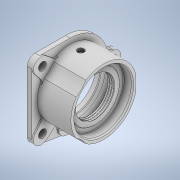
# Autodesk Inventor part: 72. Крышка подшипника
Saved by Autodesk Inventor 2021 (Build 250183000, 183)
## iProperties
Created: 2021-03-26
Part Number: 72. Крышка подшипника
Material: Типовые
Document SubType Name: Modeling
Designer: Данил
Density: 1 g/cm^3
Appearance: По умолчанию
Author: Данил
Autodesk Inventor part; units mm, degrees
ref_plane "XY Plane" through (0, 0, 0) normal (0, 0, 1) x (1, 0, 0)
sketch "Эскиз1" plane through (0, 0, 0) normal (0, 0, 1) x (1, 0, 0)
  line L0 (-25, 0) -> (25, 0)
  line L1 (25, -43) -> (25, -39.1547)
  line L2 (23, -38) -> (13.8, -38)
  line L3 (25, -43) -> (-15.3397, -43)
  line L4 (23, -38) -> (25, -39.1547)
  line L5 (13, -37.2) -> (13, -31.5)
  line L6 (13, -31.5) -> (14, -31.5)
  line L7 (14, -31.5) -> (14, -25.5)
  line L8 (14, -25.5) -> (5, -25.5)
  arc A0 (13, -37.2) -> (13.8, -38) centre (13.8, -37.2) ccw
  line L9 (5, -25.5) -> (5, -35)
  line L10 (2, -38) -> (-11, -38)
  arc A1 (2, -38) -> (5, -35) centre (2, -35) ccw
  line L11 (-14, -35) -> (-20, -35)
  line L12 (-20.5, -35.5) -> (-20.5, -39.5)
  line L13 (-21, -40) -> (-23, -40)
  arc A2 (-21, -40) -> (-20.5, -39.5) centre (-21, -39.5) ccw
  arc A3 (-20, -35) -> (-20.5, -35.5) centre (-20, -35.5) ccw
  line L14 (-23, -40) -> (-23, -43)
  line L15 (-23.5, -43.5) -> (-25, -43.5)
  arc A4 (-23.5, -43.5) -> (-23, -43) centre (-23.5, -43) ccw
  arc A5 (-14, -35) -> (-11, -38) centre (-11, -35) ccw
  point P0 (0, 0)
  point P1 (0, 0)
  point P2 (25, -38)
  dimension "d0" = 50
  dimension "d1" = 86
  dimension "d2" = 2
  dimension "d3" = 30
  dimension "d4" = 76
  dimension "d5" = 0.8
  dimension "d6" = 11
  dimension "d7" = 1
  dimension "d8" = 63
  dimension "d9" = 51
  dimension "d10" = 30
  dimension "d11" = 3
  dimension "d12" = 76
  dimension "d16" = 4.5
  dimension "d17" = 0.5
  dimension "d18" = 0.5
  dimension "d19" = 80
  dimension "d20" = 87
  dimension "d21" = 2
  dimension "d22" = 70
  dimension "d23" = 3
  dimension "d24" = 11
  constraints: 32 end point, 12 point on circle, 10 tangent, 6 centre point, 6 perpendicular, 5 vertical, 4 horizontal, 3 vertical alignment, 2 point on line, 1 coincident, 1 equal radius, 1 midpoint
  measures "d0" distance of L0.start L0.end
  measures "d1" diameter of L3 L0
  measures "d2" distance of L2.start point (25, -38)
  measures "d3" angle of L2 L4
  measures "d4" diameter of L2 L0
  measures "d5" radius of A0
  measures "d6" distance from line of L0.end L7
  measures "d7" distance between parallel lines of L7 L5
  measures "d8" diameter of L6 L0
  measures "d9" diameter of L8 L0
  measures "d10" distance from line of L0.start L9
  measures "d11" radius of A1
  measures "d12" diameter of L10 L0
  measures "d16" distance from line of L0.start L12
  measures "d17" radius of A2
  measures "d18" radius of A4
  measures "d19" diameter of L13 L0
  measures "d20" diameter of L15 L0
  measures "d21" distance from line of L0.start L14
  measures "d22" diameter of L11 L0
  measures "d23" radius of A5
  measures "d24" horizontal distance of L0.start L11.start
ref_plane "РабПлоскость1" through (-25, 0, 0) normal (1, 0, 0) x (0, 1, 0)
sketch "Эскиз2" plane through (-25, 0, 0) normal (1, 0, 0) x (0, 1, 0)
  circle A0 centre (0, 0) radius 54 construction
  arc A1 (16.522, -47.1914) -> (9.9132, -55.3148) centre (19.8264, -56.6296) ccw
  arc A2 (-9.9132, -55.3148) -> (9.9132, -55.3148) centre (0, -54) ccw
  arc A3 (-9.9132, -55.3148) -> (-16.522, -47.1914) centre (-19.8264, -56.6296) ccw
  circle A4 centre (0, -54) radius 5.25
  line L0 (50, 0) -> (50, 40)
  arc A5 (50, 40) -> (40, 50) centre (40, 40) ccw
  line L1 (40, 50) -> (-40, 50)
  line L2 (0, 0) -> (40, 40) construction
  line L3 (0, 0) -> (0, 54) construction
  circle A6 centre (38.1838, 38.1838) radius 5.25
  arc A7 (16.522, -47.1914) -> (50, 0) centre (0, 0) ccw
  arc A8 (-40, 50) -> (-49.8662, 41.6305) centre (-40, 40) ccw
  line L4 (0, 0) -> (-40, 40) construction
  circle A9 centre (-38.1838, 38.1838) radius 5.25
  line L5 (-49.8662, 41.6305) -> (-55.4149, 8.0564)
  arc A10 (-55.4149, 8.0564) -> (-54.7664, 2.1552) centre (-44.5621, 6.2628) ccw
  line L6 (-54.7664, 2.1552) -> (-46.3832, -18.6708)
  line L7 (0, 0) -> (-54, 0) construction
  line L8 (0, 0) -> (-44.5621, 6.2628) construction
  arc A11 (-46.3832, -18.6708) -> (-16.522, -47.1914) centre (0, 0) ccw
  circle A12 centre (0, 0) radius 45 construction
  dimension "d44" = 90
  dimension "d28" = 108
  dimension "d29" = 10
  dimension "d30" = 10.5
  dimension "d32" = 10
  dimension "d33" = 45
  dimension "d34" = 10.5
  dimension "d35" = 50
  dimension "d37" = 45
  dimension "d38" = 10.5
  dimension "d39" = 11
  dimension "d40" = 10
  dimension "d41" = 8
  dimension "d43" = 50
  constraints: 21 point on circle, 18 end point, 12 centre point, 12 tangent, 4 coincident, 2 equal radius, 2 point on line, 2 vertical alignment, 1 horizontal, 1 perpendicular, 1 vertical, 3 other
  measures "d28" diameter of A0
  measures "d29" radius of A2
  measures "d30" diameter of A4
  measures "d32" radius of A5
  measures "d33" angle of L3 L2
  measures "d34" diameter of A6
  measures "d35" radius of A7
  measures "d37" angle of L4 L3
  measures "d38" diameter of A9
  measures "d39" radius of A10
  measures "d40" radius of A8
  measures "d41" angle of L8 L7
  measures "d43" radius of A11
extrude "Выдавливание1" add sketch "Эскиз2" along normal blind 6
sketch "Эскиз3" plane through (-19, 0, 0) normal (1, 0, 0) x (0, 0, -1)
  arc A0 (55.3148, -9.9132) -> (55.3148, 9.9132) centre (54, 0) ccw projected
  arc A1 (55.3148, -9.9132) -> (47.1914, -16.522) centre (56.6296, -19.8264) ccw projected
  circle A2 centre (0, 0) radius 43
  line L0 (55.3148, 9.9132) -> (41.3595, 11.7641)
  line L1 (55.3148, -9.9132) -> (41.3595, -11.7641)
  arc A3 (-50, -40) -> (-41.6305, -49.8662) centre (-40, -40) ccw projected
  arc A4 (-47.8134, -33.759) -> (-33.759, -47.8134) centre (-40, -40) ccw
  line L2 (-33.759, -47.8134) -> (-20.9272, -37.564)
  line L3 (-47.8134, -33.759) -> (-37.564, -20.9272)
  line L4 (-37.564, -20.9272) -> (-20.9272, -37.564) construction
  line L5 (0, 0) -> (0, -43) construction
  line L6 (0, 0) -> (-29.2456, -29.2456) construction
  arc A5 (-40, 50) -> (-50, 40) centre (-40, 40) ccw projected
  arc A6 (-33.759, 47.8134) -> (-47.8134, 33.759) centre (-40, 40) ccw
  line L7 (-33.759, 47.8134) -> (-20.9272, 37.564)
  line L8 (-47.8134, 33.759) -> (-37.564, 20.9272)
  line L9 (-37.564, 20.9272) -> (-20.9272, 37.564) construction
  line L10 (0, 0) -> (-29.2456, 29.2456) construction
  circle A7 centre (-38.1838, 38.1838) radius 5.25 projected
  circle A8 centre (54, 0) radius 5.25 projected
  circle A9 centre (-38.1838, -38.1838) radius 5.25 projected
  arc A10 (-8.0564, -55.4149) -> (-2.1552, -54.7664) centre (-6.2628, -44.5621) ccw projected
  arc A11 (-17.2628, -44.5621) -> (4.4747, -42.1733) centre (-6.2628, -44.5621) ccw
  line L11 (-17.2628, -44.5621) -> (-17.2628, -39.3827)
  point P0 (-41.6305, -49.8662)
  point P1 (-5.0612, -55.4962)
  point P2 (-8.0564, -55.4149)
  point P3 (-2.1552, -54.7664)
  point P4 (4.5877, -42.7546)
  dimension "d47" = 86
  dimension "d48" = 45
  dimension "d49" = 23.528
  dimension "d50" = 90
  dimension "d51" = 23.528
  constraints: 24 end point, 8 point on circle, 7 tangent, 4 coincident, 3 centre point, 2 concentric, 2 midpoint, 2 vertical, 10 other
  measures "d48" angle of L5 L6
  measures "d49" distance of L3.end L2.end
  measures "d50" angle of L6 L10
  measures "d51" distance of L8.end L7.end
extrude "Выдавливание2" add sketch "Эскиз3" along normal blind 2 contours L1 A2 L0 A0 | A11 A10 L11 A2 | A2 L8 A6 A5 L7 | L2 A4 A3 L3 A2
sketch "Эскиз4" plane through (0, 0, 0) normal (0, 0, 1) x (1, 0, 0)
  line L0 (-25, 0) -> (25, 0)
  line L1 (25, -43) -> (-23, -43)
  line L2 (25, -43) -> (25, -39.1547)
  line L3 (25, -39.1547) -> (23, -38)
  line L4 (23, -38) -> (13.8, -38)
  line L5 (13, -37.2) -> (13, -32.3)
  line L6 (13.8, -31.5) -> (14, -31.5)
  line L7 (14, -31.5) -> (14, -25.5)
  line L8 (14, -25.5) -> (5, -25.5)
  arc A0 (13, -37.2) -> (13.8, -38) centre (13.8, -37.2) ccw
  arc A1 (13.8, -31.5) -> (13, -32.3) centre (13.8, -32.3) ccw
  line L9 (5, -25.5) -> (5, -35)
  line L10 (2, -38) -> (-11, -38)
  line L11 (-14, -35) -> (-14, -35)
  arc A2 (2, -38) -> (5, -35) centre (2, -35) ccw
  arc A3 (-13.9047, -35.75) -> (-11, -38) centre (-11, -35) ccw
  line L12 (-14.873, -35) -> (-20.5, -35)
  arc A4 (-13.9047, -35.75) -> (-14.873, -35) centre (-14.873, -36) ccw
  line L13 (-20.5, -35) -> (-20.5, -39.5)
  line L14 (-21, -40) -> (-23, -40)
  arc A5 (-21, -40) -> (-20.5, -39.5) centre (-21, -39.5) ccw
  line L15 (-23, -40) -> (-23, -43)
  line L16 (-23.5, -43.5) -> (-25, -43.5)
  arc A6 (-23.5, -43.5) -> (-23, -43) centre (-23.5, -43) ccw
  point P0 (0, 0)
  point P1 (0, 0)
  dimension "d54" = 50
  dimension "d55" = 86
  dimension "d56" = 30
  dimension "d57" = 2
  dimension "d58" = 76
  dimension "d59" = 51
  dimension "d60" = 1
  dimension "d61" = 11
  dimension "d62" = 0.8
  dimension "d63" = 63
  dimension "d64" = 30
  dimension "d65" = 3
  dimension "d66" = 76
  dimension "d67" = 11
  dimension "d68" = 70
  dimension "d69" = 1
  dimension "d70" = 4.5
  dimension "d71" = 0.5
  dimension "d72" = 80
  dimension "d73" = 87
  dimension "d74" = 0.5
  dimension "d75" = 2
  constraints: 34 end point, 15 point on circle, 14 tangent, 7 centre point, 6 perpendicular, 5 horizontal, 5 vertical, 2 coincident, 2 equal radius, 2 vertical alignment, 1 midpoint, 1 point on line
  measures "d54" distance of L0.start L0.end
  measures "d55" diameter of L1.start L0
  measures "d56" angle of L4 L3
  measures "d57" horizontal distance of L3.end L2.end
  measures "d58" diameter of L4 L0
  measures "d59" diameter of L8 L0
  measures "d60" distance between parallel lines of L7 L5
  measures "d61" distance from line of L0.end L7
  measures "d62" radius of A0
  measures "d63" diameter of L6 L0
  measures "d64" horizontal distance of L0.start L8.end
  measures "d65" radius of A2
  measures "d66" diameter of L10 L0
  measures "d67" distance from line of L0.start L11
  measures "d68" diameter of L12 L0
  measures "d69" radius of A4
  measures "d70" distance from line of L0.start L13
  measures "d71" radius of A5
  measures "d72" diameter of L14.end L0
  measures "d73" diameter of L16.end L0
  measures "d74" radius of A6
  measures "d75" distance from line of L16.end L15
revolve "Вращение1" add sketch "Эскиз4" angle 360 about axis through (-25, 0, 0) along (1, 0, 0)
sketch "Эскиз5" plane through (0, 0, 0) normal (0, 0, 1) x (1, 0, 0)
  line L0 (-23.5, -43.5) -> (-25, -43.5) projected
  arc A0 (-23.5, -43.5) -> (-23, -43) centre (-23.5, -43) ccw projected
  line L1 (-23, -40) -> (-23, -43) projected
  line L2 (-21, -40) -> (-23, -40) projected
  arc A1 (-21, -40) -> (-20.5, -39.5) centre (-21, -39.5) ccw projected
  line L3 (-20.5, -35) -> (-20.5, -39.5) projected
  line L4 (-14.873, -35) -> (-20.5, -35) projected
  line L5 (-25, 0) -> (25, 0) projected
  line L6 (-25, -43.5) -> (-25, 0)
  line L7 (-25, 5.25) -> (-25, -5.25) projected
  line L8 (-14.873, -35) -> (-14.873, 0)
  line L9 (-14.873, 35) -> (-14.873, -35) projected
  point P0 (0, 0)
  constraints: 4 end point, 1 collinear, 1 midpoint
revolve "Вращение2" cut sketch "Эскиз5" angle 360 about axis through (-25, 0, 0) along (1, 0, 0)
fillet "Сопряжение1" radius 6 2 edges at (-17, -42.086, 8.8189) (-17, -42.9386, -2.2971)
fillet "Сопряжение2" radius 6 2 edges at (-18, 20.9272, 37.564) (-18, 37.564, 20.9272)
fillet "Сопряжение3" radius 6 2 edges at (-18, 11.7641, -41.3595) (-18, -11.7641, -41.3595)
fillet "Сопряжение4" radius 6 2 edges at (-18, -37.564, 20.9272) (-18, -20.9272, 37.564)
sketch "Эскиз6" plane through (25, 0, 0) normal (1, 0, 0) x (0, 0, -1)
  arc A0 (-36.0961, 23.3682) -> (-23.3682, 36.0961) centre (-53.6487, 53.6487) ccw
  circle A1 centre (0, 0) radius 43 projected
  line L0 (0, 0) -> (-53.6487, 53.6487) construction
  line L1 (0, 0) -> (-43, 0) construction
  point P0 (0, 0)
  dimension "d82" = 35
  dimension "d83" = 45
  dimension "d84" = 18
  constraints: 5 point on circle, 4 end point, 1 centre point, 1 horizontal
  measures "d82" radius of A0
  measures "d83" angle of L1 L0
  measures "d84" distance of A0.end A0.start
extrude "Выдавливание3" cut sketch "Эскиз6" against normal up to surface (42 mm away) contours A1 A0 picked at (-28.727, 30.1505)
pattern_circular "Круговой массив1" count 2 over 90 about axis through (1, 0, 0) along (1, 0, 0) of "Выдавливание3"
pattern_circular "Круговой массив2" count 2 over 135 about axis through (1, 0, 0) along (-1, 0, 0) of "Выдавливание3"
ref_plane "РабПлоскость3" through (5, 25.5, 0) normal (0.0187208, 0, -0.9998247) x (0, 1, 0)
sketch "Эскиз8" plane through (5, 25.5, 0) normal (0.0187208, 0, -0.9998247) x (0, 1, 0)
  line L0 (0, -1) -> (0.4804, 0.4762)
  line L1 (0.1, 1) -> (0, 1)
  arc A0 (0.4804, 0.4762) -> (0.1, 1) centre (0.1, 0.6) ccw
  line L2 (0, 1) -> (0, -1)
  point P0 (-25.5, -4.9991)
  point P1 (0, 0)
  point P2 (0, 0)
  dimension "d98" = 0.4
  dimension "d99" = 2
  dimension "d100" = 0.1
  constraints: 6 end point, 2 point on circle, 2 tangent, 1 centre point, 1 coincident, 1 horizontal, 1 midpoint, 1 vertical
  measures "d98" radius of A0
  measures "d99" distance of L1.end L0.start
  measures "d100" horizontal distance of A0.centre L1.end
sketch3d "3D эскиз1"
  helix H0 starts at (5, 25.5, 0) axis through (5, 0, 0) along (1, 0, 0) pitch 3 turns 3 hand left
sweep "Сдвиг1" cut profiles "Эскиз8" path "3D эскиз1"
sketch "Эскиз9" plane through (-25, 0, 0) normal (-1, 0, 0) x (0, 0, 1)
  arc A0 (-3.8683, -48.8471) -> (17.1825, -45.8886) centre (6.2628, -44.5621) ccw projected
  circle A1 centre (0, 0) radius 35
  arc A2 (0.3212, -45.3971) -> (12.2044, -43.727) centre (6.2628, -44.5621) ccw
  circle A3 centre (0, 0) radius 35 projected
  line L0 (0.3212, -45.3971) -> (-0.0881, -42.4852)
  line L1 (12.2044, -43.727) -> (11.7952, -40.8151)
  arc A4 (-0.0881, -42.4852) -> (-7.7706, -34.1265) centre (-9.9907, -43.8769) ccw
  arc A5 (16.8761, -30.6626) -> (11.7952, -40.8151) centre (21.6978, -39.4234) ccw
  line L2 (0, 0) -> (6.2628, -44.5621) construction
  line L3 (-7.7706, -34.1265) -> (16.8761, -30.6626) construction
  point P0 (4.5528, -32.3946)
  point P1 (16.8761, -30.6626)
  point P2 (-7.7706, -34.1265)
  dimension "d103" = 70
  dimension "d104" = 6
  dimension "d105" = 10
  constraints: 8 end point, 8 point on circle, 6 tangent, 4 centre point, 2 coincident, 1 equal radius, 1 midpoint, 1 parallel, 1 point on line
  measures "d103" diameter of A1
  measures "d104" radius of A2
  measures "d105" radius of A4
extrude "Выдавливание4" cut sketch "Эскиз9" against normal up to surface (4.5 mm away) contours A1 A5 L1 A2 L0 A4
ref_plane "РабПлоскость4" through (0, 43, 0) normal (0, 1, 0) x (-1, 0, 0)
sketch "Эскиз10" plane through (0, 43, 0) normal (0, 1, 0) x (-1, 0, 0)
  line L0 (25, 43.5) -> (25, -43.5) projected
  point P0 (0, 0)
  point P1 (5, 0)
  point P2 (25, 0.0546)
  point P3 (25, 11.9378)
  dimension "d109" = 20
  constraints: 1 horizontal alignment
  measures "d109" distance from line of L0 point (5, 0)
hole "Отверстие1" at (-5, 43, 0) direction (0, -1, 0) diameter 8 depth 11.9 taper from width 8.4473 to width 7.985 over 7.4
